nixal_reprap4040_spoolHolderBearing (Autodesk Fusion 360 design; units mm, degrees)
Autodesk Fusion 360 part; units mm, degrees
sketch "Sketch1" plane through (0, 0, 0) normal (0, 1, 0) x (1, 0, 0)
  line L0 (0, 0) -> (32, 0)
  line L1 (32, 0) -> (32, 32)
  line L2 (32, 32) -> (0, 32)
  line L3 (0, 32) -> (0, 0)
  line L4 (3.5, 15) -> (28.5, 15)
  line L5 (28.5, 15) -> (28.5, 32)
  line L6 (28.5, 32) -> (3.5, 32)
  line L7 (3.5, 32) -> (3.5, 15)
  line L8 (5, 25) -> (5, 32)
  line L9 (27, 25) -> (27, 32)
  arc A0 (5, 25) -> (27, 25) centre (16, 25) ccw
  line L10 (12.0048, 24.8035) -> (12, 32)
  line L11 (20, 25.0187) -> (20, 32)
  arc A1 (12.0046, 25.1912) -> (20, 25.0187) centre (16, 25) ccw
  line L12 (23, 2.8972) -> (9, 2.8972)
  line L13 (9, 2.8972) -> (9, 10.3972)
  line L14 (9, 10.3972) -> (23, 10.3972)
  line L15 (23, 10.3972) -> (23, 2.8972)
  line L16 (23, 2.8972) -> (9, 10.3972) construction
  line L17 (9, 2.8972) -> (23, 10.3972) construction
  dimension "d1" = 32
  dimension "d2" = 32
  dimension "d4" = 25
  dimension "d5" = 8
  dimension "d11" = 25
  dimension "d12" = 3.5
  dimension "d16" = 22
  dimension "d17" = 7
  dimension "d20" = 14
  dimension "d21" = 7.5
  constraint horizontal L0
  constraint vertical L1
  constraint horizontal L2
  constraint vertical L3
  constraint coincident L0.start L3.end
  constraint horizontal L4
  constraint vertical L5
  constraint horizontal L6
  constraint vertical L7
  constraint coincident L2 L0.start
  constraint coincident L6 L0.start
  constraint coincident L0.start A1
  constraint coincident L10 L0.start
  constraint perpendicular L12 L13
  constraint parallel L12 L14
  constraint parallel L13 L15
  constraint horizontal L12
  constraint coincident L16 L0.start
  constraint coincident L17 L0.start
  measures "d5" diameter of A1
  measures "d12" distance of L3 L7
  measures "d16" diameter of A0
extrude "Extrude1" add sketch "Sketch1" along normal blind 20 contours L0 L1 L2 L3 L4 L5 L7 A0 | L2 L4 L6 L7 L8 A0 | L2 L4 L5 L6 L9 A0 | L2 L4 L6 L8 L9 A0 L10 L11 A1 | L2 L6 L10 L11 A1 | L4 A0 | L10 A1 | L12 L13 L14 L15
extrude "Extrude3" cut sketch "Sketch1" along normal blind 14 and the other way blind -6 contours L2 L4 L6 L8 L9 A0 L10 L11 A1 | L2 L6 L10 L11 A1 | L4 A0 | L10 A1
extrude "Extrude4" cut sketch "Sketch1" along normal blind 25 contours L2 L6 L10 L11 A1
extrude "Extrude5" cut sketch "Sketch1" along normal blind 27 contours L12 L13 L14 L15
sketch "Sketch2" plane through (0, 0, 0) normal (0, 0, 1) x (1, 0, 0)
  line L0 (0, 0) -> (32, 0)
  line L1 (32, 0) -> (32, 20)
  line L2 (32, 20) -> (0, 20)
  line L3 (0, 20) -> (0, 0)
  circle A0 centre (16, 10) radius 4.15
  dimension "d24" = 8.3
  measures "d24" diameter of A0
extrude "Extrude6" cut sketch "Sketch2" against normal blind 12 contours A0
